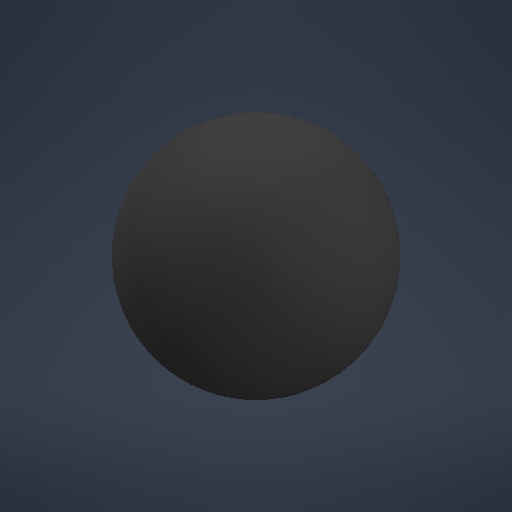
# Autodesk Inventor part: Yellow_dot_squash_ball,Trebuchet
Saved by Autodesk Inventor 2026.2 (Build 302298010, 298A)
## iProperties
Created: 2026-02-16
Part Number: Yellow_dot_squash_ball,Trebuchet
Material: Rubber
Document SubType Name: Modeling
Designer: 4aida
Mass: 22.606 g
Surface Area: 71.5026 cm^2
Volume: 24.3075 cm^3
Density: 0.93 g/cm^3
Appearance: Rubber - Black
Author: 4aida
Autodesk Inventor part; units mm, degrees
ref_plane "YZ Plane" through (0, 0, 0) normal (1, 0, 0) x (0, 1, 0)
ref_plane "XZ Plane" through (0, 0, 0) normal (0, 1, 0) x (-1, 0, 0)
ref_plane "XY Plane" through (0, 0, 0) normal (0, 0, 1) x (1, 0, 0)
sketch "Sketch1" plane through (0, 0, 0) normal (0, 0, 1) x (1, 0, 0)
  arc A0 (0, 20) -> (0, -20) centre (0, 0) ccw
  line L0 (0, 20) -> (0, -20)
  arc A1 (0, 13) -> (0, -13) centre (0, 0) ccw
  dimension "d0" = 40
  dimension "d1" = 13
  constraints: 4 point on circle, 2 centre point, 2 coincident, 2 end point, 2 point on line, 2 vertical alignment, 1 midpoint, 1 vertical
  measures "d0" diameter of A0
  measures "d1" radius of A1
revolve "Revolution1" add sketch "Sketch1" angle 360 about axis through (0, 20, 0) along (0, -1, 0) contours L0 A1 A0
body "Solid1"
